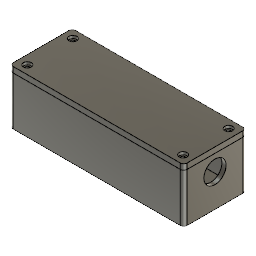
Kanssi_v1 (Autodesk Fusion 360 design; units mm, degrees)
Autodesk Fusion 360 part; units mm, degrees
sketch "Sketch1" plane through (0, 0, 0) normal (0, 0, 1) x (1, 0, 0) in component "Laatikko"
  line L0 (62.5, 22.5) -> (-62.5, 22.5)
  line L1 (-62.5, 22.5) -> (-62.5, -22.5)
  line L2 (-62.5, -22.5) -> (62.5, -22.5)
  line L3 (62.5, -22.5) -> (62.5, 22.5)
  line L4 (62.5, 22.5) -> (-62.5, -22.5) construction
  line L5 (-62.5, 22.5) -> (62.5, -22.5) construction
  dimension "d1" = 125
  dimension "d2" = 45
  constraint perpendicular L0 L1
  constraint parallel L0 L2
  constraint parallel L1 L3
  constraint horizontal L0
  constraint coincident L4 origin
  constraint coincident L5 origin
  measures "d1" distance of L1.end L2.end
  measures "d2" distance of L0.end L1.end
extrude "Extrude1" add sketch "Sketch1" along normal blind 35 makes body 1 in component "Laatikko"
sketch "Sketch2" plane through (0, 0, 35) normal (0, 0, 1) x (-1, 0, 0) in component "Laatikko"
  line L0 (-62.5, 22.5) -> (-62.5, -22.5)
  line L1 (-62.5, -22.5) -> (62.5, -22.5)
  line L2 (62.5, -22.5) -> (62.5, 22.5)
  line L3 (62.5, 22.5) -> (-62.5, 22.5)
  line L4 (-59.5, 19.5) -> (-59.5, -19.5)
  line L5 (-59.5, -19.5) -> (59.5, -19.5)
  line L6 (59.5, -19.5) -> (59.5, 19.5)
  line L7 (59.5, 19.5) -> (-59.5, 19.5)
  dimension "d5" = -3
extrude "Extrude2" cut sketch "Sketch2" against normal up to surface (32 mm away) contours L4 L5 L6 L7 bodies 1 in component "Laatikko"
fillet "Fillet1" radius 2.5 4 edges at (-62.5, -22.5, 17.5) (62.5, -22.5, 17.5) (62.5, 22.5, 17.5) (-62.5, 22.5, 17.5) on bodies 1 in component "Laatikko"
sketch "Sketch4" plane through (0, 0, 3) normal (0, 0, 1) x (-1, 0, 0) in component "Laatikko"
  line L0 (-59.5, 19.5) -> (-59.5, -19.5)
  line L1 (-59.5, -19.5) -> (59.5, -19.5)
  line L2 (59.5, -19.5) -> (59.5, 19.5)
  line L3 (59.5, 19.5) -> (-59.5, 19.5)
  circle A0 centre (21.684, -15.7) radius 1.025
  circle A1 centre (21.684, 15.415) radius 1.025
  circle A2 centre (-53.5, 15.415) radius 1.025
  dimension "d12" = 2.05
  dimension "d13" = 2.05
  dimension "d14" = 31.115
  dimension "d15" = 2.05
  dimension "d16" = 75.184
  dimension "d66" = 6
  measures "d12" diameter of A0
  measures "d13" diameter of A1
  measures "d14" distance of A0.centre A1.centre
  measures "d15" diameter of A2
  measures "d16" distance of A1.centre A2.centre
  measures "d66" distance of L0 A2.centre
extrude "Extrude3" cut sketch "Sketch4" against normal blind 6 contours A0 | A1 | A2 bodies 1 in component "Laatikko"
sketch "Sketch5" plane through (0, 0, 3) normal (0, 0, 1) x (-1, 0, 0) in component "Laatikko"
  circle A0 centre (21.684, -15.7) radius 1.025
  circle A1 centre (21.684, 15.415) radius 1.025
  circle A2 centre (-53.5, 15.415) radius 1.025
  line L0 (-59.5, 19.5) -> (-59.5, -19.5)
  line L1 (-59.5, -19.5) -> (59.5, -19.5)
  line L2 (59.5, -19.5) -> (59.5, 19.5)
  line L3 (59.5, 19.5) -> (-59.5, 19.5)
  circle A3 centre (-53.5, -15.7) radius 0.975
  dimension "d19" = 1.95
  dimension "d64" = 75.184
  dimension "d65" = 31.115
  measures "d19" diameter of A3
  measures "d64" horizontal distance of A0.centre A3.centre
  measures "d65" distance of A2.centre A3.centre
extrude "Extrude4" add sketch "Sketch5" along normal blind 5 contours A3 bodies 1 in component "Laatikko"
sketch "Sketch6" plane through (0, 0, 0) normal (0, 0, -1) x (1, 0, 0) in component "Laatikko"
  circle A0 centre (-21.684, -15.7) radius 1.025
  circle A1 centre (-21.684, 15.415) radius 1.025
  circle A2 centre (53.5, 15.415) radius 1.025
  arc A3 (-62.5, -20) -> (-60, -22.5) centre (-60, -20) ccw
  line L0 (-60, -22.5) -> (60, -22.5)
  arc A4 (60, -22.5) -> (62.5, -20) centre (60, -20) ccw
  line L1 (62.5, -20) -> (62.5, 20)
  arc A5 (62.5, 20) -> (60, 22.5) centre (60, 20) ccw
  line L2 (60, 22.5) -> (-60, 22.5)
  arc A6 (-60, 22.5) -> (-62.5, 20) centre (-60, 20) ccw
  line L3 (-62.5, 20) -> (-62.5, -20)
  circle A7 centre (-21.684, 15.415) radius 2
  circle A8 centre (-21.684, -15.7) radius 2
  circle A9 centre (53.5, 15.415) radius 2
  dimension "d23" = 4
  dimension "d24" = 4
  dimension "d25" = 4
  constraint concentric A1 A7
  constraint concentric A0 A8
  constraint concentric A2 A9
  measures "d23" diameter of A7
  measures "d24" diameter of A8
  measures "d25" diameter of A9
extrude "Extrude5" cut sketch "Sketch6" against normal blind 1.5 contours A7 | A8 | A9 bodies 1 in component "Laatikko"
sketch "Sketch7" plane through (0, 0, 35) normal (0, 0, 1) x (-1, 0, 0) in component "Laatikko"
  arc A0 (60, -22.5) -> (62.5, -20) centre (60, -20) ccw
  line L0 (62.5, -20) -> (62.5, 20)
  arc A1 (62.5, 20) -> (60, 22.5) centre (60, 20) ccw
  line L1 (60, 22.5) -> (-60, 22.5)
  arc A2 (-60, 22.5) -> (-62.5, 20) centre (-60, 20) ccw
  line L2 (-62.5, 20) -> (-62.5, -20)
  arc A3 (-62.5, -20) -> (-60, -22.5) centre (-60, -20) ccw
  line L3 (-60, -22.5) -> (60, -22.5)
  line L4 (59.5, 19.5) -> (59.5, -19.5)
  line L5 (59.5, -19.5) -> (-59.5, -19.5)
  line L6 (-59.5, -19.5) -> (-59.5, 19.5)
  line L7 (-59.5, 19.5) -> (59.5, 19.5)
  circle A4 centre (55.9674, -16.3565) radius 4.7288
  circle A5 centre (55.9674, 16.3565) radius 4.7288
  circle A6 centre (-55.9674, 16.3565) radius 4.7288
  circle A7 centre (-55.9674, -16.3565) radius 4.7288
  constraint coincident L4.end A4
  constraint coincident L4.start A5
  constraint coincident L6.end A6
  constraint coincident L5.end A7
extrude "Extrude6" add sketch "Sketch7" against normal blind 11 contours L4 L7 A5 | L4 L5 A4 | L6 L7 A6 | L5 L6 A7 bodies 1 in component "Laatikko"
fillet "Fillet2" radius 1.5 8 edges at (52.4348, -19.5, 29.5) (59.5, -13.2129, 29.5) (52.4348, 19.5, 29.5) (59.5, 13.2129, 29.5) (-52.4348, 19.5, 29.5) (-59.5, 13.2129, 29.5) (-52.4348, -19.5, 29.5) (-59.5, -13.2129, 29.5) on bodies 1 in component "Laatikko"
sketch "Sketch8" plane through (0, 0, 35) normal (0, 0, 1) x (-1, 0, 0) in component "Laatikko"
  arc A0 (60, -22.5) -> (62.5, -20) centre (60, -20) ccw
  line L0 (62.5, -20) -> (62.5, 20)
  arc A1 (62.5, 20) -> (60, 22.5) centre (60, 20) ccw
  line L1 (60, 22.5) -> (-60, 22.5)
  arc A2 (-60, 22.5) -> (-62.5, 20) centre (-60, 20) ccw
  line L2 (-62.5, 20) -> (-62.5, -20)
  arc A3 (-62.5, -20) -> (-60, -22.5) centre (-60, -20) ccw
  line L3 (-60, -22.5) -> (60, -22.5)
  line L4 (59.5, 10.4687) -> (59.5, -10.4687)
  arc A4 (57.5105, -11.8866) -> (59.5, -10.4687) centre (58, -10.4687) ccw
  arc A5 (57.5105, -11.8866) -> (51.4062, -17.6042) centre (55.9674, -16.3565) ccw
  arc A6 (49.9594, -19.5) -> (51.4062, -17.6042) centre (49.9594, -18) ccw
  line L5 (49.9594, -19.5) -> (-49.9594, -19.5)
  arc A7 (-51.4062, -17.6042) -> (-49.9594, -19.5) centre (-49.9594, -18) ccw
  arc A8 (-51.4062, -17.6042) -> (-57.5105, -11.8866) centre (-55.9674, -16.3565) ccw
  arc A9 (-59.5, -10.4687) -> (-57.5105, -11.8866) centre (-58, -10.4687) ccw
  line L6 (-59.5, -10.4687) -> (-59.5, 10.4687)
  arc A10 (-57.5105, 11.8866) -> (-59.5, 10.4687) centre (-58, 10.4687) ccw
  arc A11 (-57.5105, 11.8866) -> (-51.4062, 17.6042) centre (-55.9674, 16.3565) ccw
  arc A12 (-49.9594, 19.5) -> (-51.4062, 17.6042) centre (-49.9594, 18) ccw
  line L7 (-49.9594, 19.5) -> (49.9594, 19.5)
  arc A13 (51.4062, 17.6042) -> (49.9594, 19.5) centre (49.9594, 18) ccw
  arc A14 (51.4062, 17.6042) -> (57.5105, 11.8866) centre (55.9674, 16.3565) ccw
  arc A15 (59.5, 10.4687) -> (57.5105, 11.8866) centre (58, 10.4687) ccw
  circle A16 centre (-55.9674, -16.3565) radius 1.5
  circle A17 centre (-55.9674, 16.3565) radius 1.5
  circle A18 centre (55.9674, 16.3565) radius 1.5
  circle A19 centre (55.9674, -16.3565) radius 1.5
  dimension "d37" = 3
  dimension "d38" = 3
  dimension "d39" = 3
  dimension "d40" = 3
  constraint concentric A8 A16
  constraint concentric A11 A17
  constraint concentric A14 A18
  constraint concentric A5 A19
  measures "d37" diameter of A16
  measures "d38" diameter of A17
  measures "d39" diameter of A18
  measures "d40" diameter of A19
extrude "Extrude7" cut sketch "Sketch8" against normal blind 9 contours A16 | A17 | A18 | A19 bodies 1 in component "Laatikko"
sketch "Sketch1 (2)" plane through (0, 0, 35) normal (0, 0, 1) x (-1, 0, 0) in component "Kansi"
  circle A0 centre (-55.9674, 16.3565) radius 1.5
  circle A1 centre (55.9674, 16.3565) radius 1.5
  circle A2 centre (-55.9674, -16.3565) radius 1.5
  circle A3 centre (55.9674, -16.3565) radius 1.5
  arc A4 (60, -22.5) -> (62.5, -20) centre (60, -20) ccw
  line L0 (62.5, -20) -> (62.5, 20)
  arc A5 (62.5, 20) -> (60, 22.5) centre (60, 20) ccw
  line L1 (60, 22.5) -> (-60, 22.5)
  arc A6 (-60, 22.5) -> (-62.5, 20) centre (-60, 20) ccw
  line L2 (-62.5, 20) -> (-62.5, -20)
  arc A7 (-62.5, -20) -> (-60, -22.5) centre (-60, -20) ccw
  line L3 (-60, -22.5) -> (60, -22.5)
  line L4 (59.5, 10.4687) -> (59.5, -10.4687)
  arc A8 (57.5105, -11.8866) -> (59.5, -10.4687) centre (58, -10.4687) ccw
  arc A9 (57.5105, -11.8866) -> (51.4062, -17.6042) centre (55.9674, -16.3565) ccw
  arc A10 (49.9594, -19.5) -> (51.4062, -17.6042) centre (49.9594, -18) ccw
  line L5 (49.9594, -19.5) -> (-49.9594, -19.5)
  arc A11 (-51.4062, -17.6042) -> (-49.9594, -19.5) centre (-49.9594, -18) ccw
  arc A12 (-51.4062, -17.6042) -> (-57.5105, -11.8866) centre (-55.9674, -16.3565) ccw
  arc A13 (-59.5, -10.4687) -> (-57.5105, -11.8866) centre (-58, -10.4687) ccw
  line L6 (-59.5, -10.4687) -> (-59.5, 10.4687)
  arc A14 (-57.5105, 11.8866) -> (-59.5, 10.4687) centre (-58, 10.4687) ccw
  arc A15 (-57.5105, 11.8866) -> (-51.4062, 17.6042) centre (-55.9674, 16.3565) ccw
  arc A16 (-49.9594, 19.5) -> (-51.4062, 17.6042) centre (-49.9594, 18) ccw
  line L7 (-49.9594, 19.5) -> (49.9594, 19.5)
  arc A17 (51.4062, 17.6042) -> (49.9594, 19.5) centre (49.9594, 18) ccw
  arc A18 (51.4062, 17.6042) -> (57.5105, 11.8866) centre (55.9674, 16.3565) ccw
  arc A19 (59.5, 10.4687) -> (57.5105, 11.8866) centre (58, 10.4687) ccw
  line L8 (-60, -22.5) -> (60, -22.5)
  line L9 (-62.5, 20) -> (-62.5, -20)
  arc A20 (-60, 22.5) -> (-62.5, 20) centre (-60, 20) ccw
  line L10 (60, 22.5) -> (-60, 22.5)
  line L11 (62.5, -20) -> (62.5, 20)
  arc A21 (60, -22.5) -> (62.5, -20) centre (60, -20) ccw
  circle A22 centre (-55.9674, -16.3565) radius 1.55
  circle A23 centre (-55.9674, 16.3565) radius 1.55
  circle A24 centre (55.9674, 16.3565) radius 1.55
  circle A25 centre (55.9674, -16.3565) radius 1.55
  arc A26 (-62.5, -20) -> (-60, -22.5) centre (-60, -20) ccw
  arc A27 (62.5, 20) -> (60, 22.5) centre (60, 20) ccw
  dimension "d43" = 3.1
  dimension "d44" = 3.1
  dimension "d45" = 3.1
  dimension "d46" = 3.1
  constraint concentric A2 A22
  constraint concentric A0 A23
  constraint concentric A1 A24
  constraint concentric A3 A25
  measures "d43" diameter of A22
  measures "d44" diameter of A23
  measures "d45" diameter of A24
  measures "d46" diameter of A25
extrude "Extrude1'" add sketch "Sketch1 (2)" along normal blind 4 separate body contours A4 L0 A5 L1 A6 L2 A7 L3 L8 L9 A20 L10 L11 A21 A26 A27 | L4 A8 A9 A10 L5 A11 A12 A13 L6 A14 A15 A16 L7 A17 A18 A19 makes body 2 in component "Kansi"
sketch "Sketch2 (2)" plane through (0, 0, 39) normal (0, 0, 1) x (-1, 0, 0) in component "Kansi"
  arc A0 (60, -22.5) -> (62.5, -20) centre (60, -20) ccw
  line L0 (62.5, -20) -> (62.5, 20)
  arc A1 (62.5, 20) -> (60, 22.5) centre (60, 20) ccw
  line L1 (60, 22.5) -> (-60, 22.5)
  arc A2 (-60, 22.5) -> (-62.5, 20) centre (-60, 20) ccw
  line L2 (-62.5, 20) -> (-62.5, -20)
  arc A3 (-62.5, -20) -> (-60, -22.5) centre (-60, -20) ccw
  line L3 (-60, -22.5) -> (60, -22.5)
  circle A4 centre (55.9674, 16.3565) radius 2.8
  circle A5 centre (55.9674, -16.3565) radius 2.8
  circle A6 centre (-55.9674, -16.3565) radius 2.8
  circle A7 centre (-55.9674, 16.3565) radius 2.8
  circle A8 centre (55.9674, -16.3565) radius 1.55
  circle A9 centre (-55.9674, 16.3565) radius 1.55
  circle A10 centre (55.9674, 16.3565) radius 1.55
  circle A11 centre (-55.9674, -16.3565) radius 1.55
  dimension "d49" = 5.6
  dimension "d50" = 5.6
  dimension "d51" = 5.6
  dimension "d52" = 5.6
  constraint concentric A5 A8
  measures "d49" diameter of A4
  measures "d50" diameter of A5
  measures "d51" diameter of A6
  measures "d52" diameter of A7
extrude "Extrude2'" cut sketch "Sketch2 (2)" against normal blind 2 contours A4 | A5 | A6 | A7 | A9 | A10 | A11 bodies 2 in component "Kansi"
sketch "Sketch9" plane through (62.5, 0, 0) normal (1, 0, 0) x (0, 1, 0) in component "Laatikko"
  line L0 (20, 0) -> (20, 35)
  line L1 (20, 35) -> (-20, 35)
  line L2 (-20, 35) -> (-20, 0)
  line L3 (-20, 0) -> (20, 0)
  circle A0 centre (0, 23.5) radius 8
  dimension "d55" = 16
  dimension "d61" = 11.5
  measures "d55" diameter of A0
  measures "d61" distance of L1 A0.centre
extrude "Extrude8" cut sketch "Sketch9" against normal blind 5 contours A0 bodies 1 in component "Laatikko"
sketch "Sketch10" plane through (-62.5, 0, 0) normal (-1, 0, 0) x (0, -1, 0) in component "Laatikko"
  line L0 (-20, 35) -> (-20, 0)
  line L1 (-20, 0) -> (20, 0)
  line L2 (20, 0) -> (20, 35)
  line L3 (20, 35) -> (-20, 35)
  circle A0 centre (0, 23.5) radius 8
  dimension "d58" = 16
  dimension "d62" = 11.5
  measures "d58" diameter of A0
  measures "d62" distance of L3 A0.centre
extrude "Extrude9" cut sketch "Sketch10" against normal blind 5 contours A0 bodies 1 in component "Laatikko"
sketch "Sketch12" plane through (0, 0, 3) normal (0, 0, 1) x (-1, 0, 0) in component "Laatikko"
  circle A0 centre (-53.5, -15.7) radius 0.975
  circle A1 centre (21.684, -15.7) radius 1.025
  circle A2 centre (21.684, 15.415) radius 1.025
  circle A3 centre (-53.5, 15.415) radius 1.025
  line L0 (-59.5, 19.5) -> (-59.5, -19.5)
  line L1 (-59.5, -19.5) -> (59.5, -19.5)
  line L2 (59.5, -19.5) -> (59.5, 19.5)
  line L3 (59.5, 19.5) -> (-59.5, 19.5)
  circle A4 centre (-53.5, -15.7) radius 2.75
  circle A5 centre (21.684, -15.7) radius 2.75
  circle A6 centre (21.684, 15.415) radius 2.75
  circle A7 centre (-53.5, 15.415) radius 2.75
  dimension "d68" = 5.5
  dimension "d85" = 5.5
  dimension "d86" = 5.5
  dimension "d87" = 5.5
  constraint concentric A0 A4
  constraint concentric A1 A5
  constraint concentric A2 A6
  constraint concentric A3 A7
  measures "d68" diameter of A4
  measures "d85" diameter of A5
  measures "d86" diameter of A6
  measures "d87" diameter of A7
extrude "Extrude10" add sketch "Sketch12" along normal blind 3 contours A4 | A5 | A6 | A7 bodies 1 in component "Laatikko"
fillet "Fillet4" radius 2.5 12 edges at (-51.1518, 18.91, 24) (-52.7347, 12.9052, 24) (-58.8706, 11.6902, 24) (-58.8706, -11.6902, 24) (-52.7347, -12.9052, 24) (-51.1518, -18.91, 24) (51.1518, -18.91, 24) (52.7347, -12.9052, 24) (58.8706, -11.6902, 24) (58.8706, 11.6902, 24) (52.7347, 12.9052, 24) (51.1518, 18.91, 24) on bodies 1 in component "Laatikko"
sketch "Sketch13" plane through (0, 0, 3) normal (0, 0, 1) x (-1, 0, 0) in component "Laatikko"
  line L0 (-59.5, 19.5) -> (-59.5, -19.5)
  line L1 (-59.5, -19.5) -> (59.5, -19.5)
  line L2 (59.5, -19.5) -> (59.5, 19.5)
  line L3 (59.5, 19.5) -> (-59.5, 19.5)
  line L4 (48.5, -19.5) -> (48.5, 5.5)
  line L5 (48.5, 5.5) -> (45.5, 5.5)
  line L6 (45.5, 5.5) -> (45.5, -19.5)
  line L7 (33, 5.5) -> (33, -19.5)
  line L8 (33, 5.5) -> (30, 5.5)
  line L9 (30, 5.5) -> (30, -19.5)
  circle A0 centre (-53.5, 15.415) radius 2.75
  circle A1 centre (21.684, 15.415) radius 2.75
  circle A2 centre (21.684, -15.7) radius 2.75
  circle A3 centre (-53.5, -15.7) radius 2.75
  dimension "d72" = 25
  dimension "d73" = 3
  dimension "d74" = 12.5
  dimension "d75" = 3
  dimension "d88" = 89.5
  constraint coincident L1 L4.start
  constraint perpendicular L1 L4
  constraint perpendicular L4 L5
  constraint coincident L1 L6.end
  constraint perpendicular L1 L6
  constraint coincident L1 L7.end
  constraint perpendicular L1 L7
  constraint perpendicular L7 L8
  constraint coincident L1 L9.end
  constraint perpendicular L1 L9
  measures "d72" distance of L4.start L4.end
  measures "d73" distance of L4.end L5.end
  measures "d74" distance of L5.end L7.start
  measures "d75" distance of L7.start L8.end
  measures "d88" distance of L0 L9
extrude "Extrude11" add sketch "Sketch13" along normal blind 8 contours L1 L7 L8 L9 | L1 L4 L5 L6 bodies 1 in component "Laatikko"
sketch "Sketch14" plane through (0, 0, 11) normal (0, 0, 1) x (-1, 0, 0) in component "Laatikko"
  line L0 (45.5, 5.5) -> (45.5, -19.5)
  line L1 (45.5, -19.5) -> (48.5, -19.5)
  line L2 (48.5, -19.5) -> (48.5, 5.5)
  line L3 (48.5, 5.5) -> (45.5, 5.5)
  line L4 (50.5, -10.3745) -> (45.5, -10.3745)
  dimension "d79" = 16
  constraint coincident L0 L4.end
  constraint perpendicular L0 L4
  measures "d79" distance of L2.end L4.start
extrude "Extrude12" add sketch "Sketch14" along normal blind 24 contours L0 L1 L2 L4 bodies 1 in component "Laatikko"
sketch "Sketch15" plane through (0, 0, 11) normal (0, 0, 1) x (-1, 0, 0) in component "Laatikko"
  line L0 (33, 5.5) -> (30, 5.5)
  line L1 (30, 5.5) -> (30, -19.5)
  line L2 (30, -19.5) -> (33, -19.5)
  line L3 (33, -19.5) -> (33, 5.5)
  line L4 (33, -13.5) -> (30, -13.5)
  dimension "d82" = 19
  constraint coincident L1 L4.end
  constraint perpendicular L1 L4
  measures "d82" distance of L0.start L4.start
extrude "Extrude13" add sketch "Sketch15" along normal blind 24 contours L1 L2 L3 L4 bodies 1 in component "Laatikko"
component "Laatikko" placed x (1, 0, 0) y (0, 1, 0) z (0, 0, 1) at (0, 0, 0)
component "Kansi" placed x (1, 0, 0) y (0, 1, 0) z (0, 0, 1) at (0, 0, 0)
